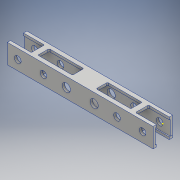
# Autodesk Inventor part: BT-BTK120-DriveFrameTube
Saved by Autodesk Inventor 2017 (Build 210142000, 142)
## iProperties
Created: 2016-09-24
Part Number: BT-BTK120-DriveFrameTube
Material: Aluminum 6061
Document SubType Name: Modeling
Designer: vslabsal
Density: 2.7 g/cm^3
Appearance: Aluminum - Flat
Author: vslabsal
Autodesk Inventor part; units mm, degrees
ref_plane "YZ Plane" through (0, 0, 0) normal (1, 0, 0) x (0, 1, 0)
ref_plane "XZ Plane" through (0, 0, 0) normal (0, 1, 0) x (-1, 0, 0)
ref_plane "XY Plane" through (0, 0, 0) normal (0, 0, 1) x (1, 0, 0)
sketch "Sketch1" plane through (0, 0, 0) normal (0, 0, 1) x (1, 0, 0)
  arc A0 (-183.6588, -17.77) -> (-179.4288, -22) centre (-179.4288, -17.77) ccw
  arc A1 (-179.9924, 22) -> (-183.6588, 16.912) centre (-179.5223, 17.7962) ccw
  line L0 (-183.6588, -17.77) -> (-183.6588, 16.912)
  line L1 (-205.2488, 21.796) -> (-205.2488, -22.654)
  line L2 (-286.5288, 24.971) -> (-208.4238, 24.971)
  line L3 (-286.5288, -25.829) -> (-208.4238, -25.829)
  line L4 (-52.9925, -22) -> (-179.4288, -22)
  line L5 (-52.4305, 22) -> (-179.9924, 22)
  arc A2 (-48.2588, 16.912) -> (-52.4305, 22) centre (-52.4009, 17.7701) ccw
  line L6 (-48.2588, -17.77) -> (-48.2588, 16.912)
  arc A3 (-52.9925, -22) -> (-48.2588, -17.77) centre (-52.4887, -17.8001) ccw
  arc A4 (-205.2488, 21.796) -> (-208.4238, 24.971) centre (-208.4238, 21.796) ccw
  arc A5 (-208.4238, -25.829) -> (-205.2488, -22.654) centre (-208.4238, -22.654) ccw
  line L7 (204.3262, -25.4) -> (282.4312, -25.4)
  line L8 (204.3262, 25.4) -> (282.4312, 25.4)
  line L9 (44.1612, -17.77) -> (44.1612, 16.912)
  arc A6 (44.1612, -17.77) -> (48.3912, -22) centre (48.3912, -17.77) ccw
  line L10 (175.3896, 22) -> (47.8276, 22)
  line L11 (174.8276, -22) -> (48.3912, -22)
  arc A7 (174.8276, -22) -> (179.5612, -17.77) centre (175.3313, -17.8001) ccw
  arc A8 (179.5612, 16.912) -> (175.3896, 22) centre (175.4192, 17.7701) ccw
  arc A9 (47.8276, 22) -> (44.1612, 16.912) centre (48.2978, 17.7962) ccw
  line L12 (179.5612, -17.77) -> (179.5612, 16.912)
  arc A10 (201.1512, -22.225) -> (204.3262, -25.4) centre (204.3262, -22.225) ccw
  arc A11 (204.3262, 25.4) -> (201.1512, 22.225) centre (204.3262, 22.225) ccw
  line L13 (201.1512, 22.225) -> (201.1512, -22.225)
  line L14 (-286.5288, 38.1) -> (282.4312, 38.1)
  line L15 (-286.5288, -38.1) -> (282.4312, -38.1)
  line L16 (282.4312, 38.1) -> (282.4312, 25.4)
  line L17 (282.4312, -25.4) -> (282.4312, -38.1)
  line L18 (-286.5288, 38.1) -> (-286.5288, 24.971)
  line L19 (-286.5288, -25.829) -> (-286.5288, -38.1)
  point P0 (0, 0)
  dimension "d0" = 135.4
  dimension "d1" = 44
  dimension "d2" = 78.105
  dimension "d3" = 50.8
  dimension "d4" = 44.45
  dimension "d5" = 21.59
  dimension "d6" = 135.4
  dimension "d7" = 44
  dimension "d8" = 78.105
  dimension "d9" = 50.8
  dimension "d10" = 568.96
  dimension "d11" = 21.59
  constraints: 40 end point, 28 point on circle, 12 centre point, 8 vertical, 7 horizontal, 2 perpendicular, 1 parallel, 1 point on line
  measures "d0" distance between parallel lines of L6 L0
  measures "d1" distance between parallel lines of L4 L5
  measures "d2" distance of L3.start L3.end
  measures "d3" distance between parallel lines of L3 L2
  measures "d4" distance of L1.start L1.end
  measures "d5" distance between parallel lines of L0 L1
  measures "d6" distance between parallel lines of L12 L9
  measures "d7" distance between parallel lines of L11 L10
  measures "d8" distance of L7.start L7.end
  measures "d9" distance between parallel lines of L7 L8
  measures "d10" distance of L14.end L14.start
  measures "d11" distance between parallel lines of L13 L12
extrude "Extrusion1" add sketch "Sketch1" along normal blind 9.525
sketch "Sketch2" plane through (-286.5288, 38.1, 0) normal (0, 1, 0) x (1, 0, 0)
  line L0 (0, 57.15) -> (568.96, 57.15)
  line L1 (568.96, 57.15) -> (568.96, 0)
  line L2 (568.96, 0) -> (0, 0)
  line L3 (0, 0) -> (0, 57.15)
  circle A0 centre (40.64, 28.575) radius 13
  circle A1 centre (140.776, 28.575) radius 13
  circle A2 centre (230.152, 28.575) radius 16
  circle A3 centre (528.32, 28.575) radius 13
  circle A4 centre (428.184, 28.575) radius 13
  circle A5 centre (338.808, 28.575) radius 16
  point P0 (286.5288, 0)
  point P1 (99.06, 38.1)
  dimension "d14" = 26
  dimension "d15" = 26
  dimension "d16" = 32
  dimension "d17" = 26
  dimension "d18" = 26
  dimension "d19" = 32
  dimension "d20" = 568.96
  dimension "d21" = 57.15
  dimension "d22" = 40.64
  dimension "d23" = 140.776
  dimension "d24" = 230.152
  dimension "d25" = 230.152
  dimension "d26" = 40.64
  dimension "d27" = 140.776
  constraints: 8 end point, 6 centre point, 2 parallel, 1 horizontal, 1 perpendicular
  measures "d14" diameter of A0
  measures "d15" diameter of A1
  measures "d16" diameter of A2
  measures "d17" diameter of A3
  measures "d18" diameter of A4
  measures "d19" diameter of A5
  measures "d20" distance between parallel lines of L1 L3
  measures "d21" distance between parallel lines of L2 L0
  measures "d22" distance from line of A0.centre L3
  measures "d23" distance from line of A1.centre L3
  measures "d24" distance from line of A2.centre L3
  measures "d25" distance from line of A5.centre L1
  measures "d26" distance from line of A3.centre L1
  measures "d27" distance from line of A4.centre L1
extrude "Extrusion2" add sketch "Sketch2" against normal blind 9.525
sketch "Sketch3" plane through (-286.5288, -38.1, 0) normal (0, -1, 0) x (1, 0, 0)
  line L0 (0, 0) -> (568.96, 0)
  line L1 (568.96, 0) -> (568.96, -57.15)
  line L2 (568.96, -57.15) -> (0, -57.15)
  line L3 (0, -57.15) -> (0, 0)
  circle A0 centre (40.64, -28.575) radius 13
  circle A1 centre (140.776, -28.575) radius 13
  circle A2 centre (230.152, -28.575) radius 16
  circle A3 centre (528.32, -28.575) radius 13
  circle A4 centre (428.184, -28.575) radius 13
  circle A5 centre (338.808, -28.575) radius 16
  point P0 (286.5288, 0)
  dimension "d30" = 26
  dimension "d31" = 26
  dimension "d32" = 32
  dimension "d33" = 26
  dimension "d34" = 26
  dimension "d35" = 32
  dimension "d36" = 568.96
  dimension "d37" = 57.15
  dimension "d38" = 40.64
  dimension "d39" = 140.776
  dimension "d40" = 230.152
  dimension "d41" = 230.152
  dimension "d42" = 40.64
  dimension "d43" = 140.776
  constraints: 8 end point, 6 centre point, 2 parallel, 1 horizontal, 1 perpendicular
  measures "d30" diameter of A0
  measures "d31" diameter of A1
  measures "d32" diameter of A2
  measures "d33" diameter of A3
  measures "d34" diameter of A4
  measures "d35" diameter of A5
  measures "d36" distance between parallel lines of L1 L3
  measures "d37" distance between parallel lines of L2 L0
  measures "d38" distance from line of A0.centre L3
  measures "d39" distance from line of A1.centre L3
  measures "d40" distance from line of A2.centre L3
  measures "d41" distance from line of A5.centre L1
  measures "d42" distance from line of A3.centre L1
  measures "d43" distance from line of A4.centre L1
extrude "Extrusion3" add sketch "Sketch3" against normal blind 9.525
sketch "Sketch5" plane through (282.4312, -38.1, -57.15) normal (0, 0, -1) x (-1, 0, 0)
  arc A0 (102.8699, 20.33) -> (107.0999, 16.1) centre (107.0999, 20.33) ccw
  arc A1 (106.5363, 60.1) -> (102.8699, 55.012) centre (107.0065, 55.8962) ccw
  line L0 (102.8699, 20.33) -> (102.8699, 55.012)
  line L1 (81.2799, 59.896) -> (81.2799, 15.446)
  line L2 (-0.0001, 63.071) -> (78.1049, 63.071)
  line L3 (0, 12.271) -> (78.105, 12.271)
  line L4 (233.5363, 16.1) -> (107.0999, 16.1)
  line L5 (234.0983, 60.1) -> (106.5363, 60.1)
  arc A2 (238.2699, 55.012) -> (234.0983, 60.1) centre (234.1279, 55.8701) ccw
  line L6 (238.2699, 20.33) -> (238.2699, 55.012)
  arc A3 (233.5363, 16.1) -> (238.2699, 20.33) centre (234.04, 20.2999) ccw
  arc A4 (81.2799, 59.896) -> (78.1049, 63.071) centre (78.1049, 59.896) ccw
  arc A5 (78.105, 12.271) -> (81.2799, 15.446) centre (78.1049, 15.446) ccw
  line L7 (490.855, 12.7) -> (568.96, 12.7)
  line L8 (490.855, 63.5) -> (568.9599, 63.5)
  line L9 (330.69, 20.33) -> (330.69, 55.012)
  arc A6 (330.69, 20.33) -> (334.92, 16.1) centre (334.92, 20.33) ccw
  line L10 (461.9184, 60.1) -> (334.3564, 60.1)
  line L11 (461.3564, 16.1) -> (334.92, 16.1)
  arc A7 (461.3564, 16.1) -> (466.09, 20.33) centre (461.8601, 20.2999) ccw
  arc A8 (466.09, 55.012) -> (461.9184, 60.1) centre (461.948, 55.8701) ccw
  arc A9 (334.3564, 60.1) -> (330.69, 55.012) centre (334.8266, 55.8962) ccw
  line L12 (466.09, 20.33) -> (466.09, 55.012)
  arc A10 (487.68, 15.875) -> (490.855, 12.7) centre (490.855, 15.875) ccw
  arc A11 (490.855, 63.5) -> (487.68, 60.325) centre (490.855, 60.325) ccw
  line L13 (487.68, 60.325) -> (487.68, 15.875)
  line L14 (-0.0001, 76.2) -> (568.9599, 76.2)
  line L15 (0, 0) -> (568.96, 0)
  line L16 (568.9599, 76.2) -> (568.9599, 63.5)
  line L17 (568.96, 12.7) -> (568.96, 0)
  line L18 (-0.0001, 76.2) -> (-0.0001, 63.071)
  line L19 (0, 12.271) -> (0, 0)
  point P0 (282.4312, 38.1)
  dimension "d60" = 135.4
  dimension "d61" = 44
  dimension "d62" = 78.105
  dimension "d63" = 50.8
  dimension "d64" = 44.45
  dimension "d65" = 21.59
  dimension "d66" = 135.4
  dimension "d67" = 44
  dimension "d68" = 78.105
  dimension "d69" = 50.8
  dimension "d70" = 568.96
  dimension "d71" = 21.59
  constraints: 40 end point, 28 point on circle, 12 centre point, 8 vertical, 7 horizontal, 2 perpendicular, 1 parallel, 1 point on line
  measures "d60" distance between parallel lines of L6 L0
  measures "d61" distance between parallel lines of L4 L5
  measures "d62" distance of L3.start L3.end
  measures "d63" distance between parallel lines of L3 L2
  measures "d64" distance of L1.start L1.end
  measures "d65" distance between parallel lines of L0 L1
  measures "d66" distance between parallel lines of L12 L9
  measures "d67" distance between parallel lines of L11 L10
  measures "d68" distance of L7.start L7.end
  measures "d69" distance between parallel lines of L7 L8
  measures "d70" distance of L14.end L14.start
  measures "d71" distance between parallel lines of L13 L12
extrude "Extrusion5" add sketch "Sketch5" along normal blind 9.525
sketch "Sketch6" plane through (282.4313, 24.971, -57.15) normal (1, 0, 0) x (0, 0, -1)
  point P0 (-57.15, -24.971)
body "Solid1"
